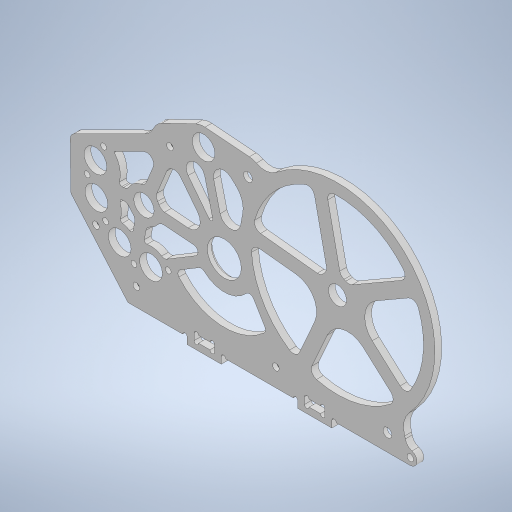
# Autodesk Inventor part: 右フレーム
Saved by Autodesk Inventor 2023 (Build 270158000, 158)
## iProperties
Created: 2022-06-19
Part Number: 右フレーム
Material: 一般
Document SubType Name: Modeling
Designer: muzho
Density: 1 g/cm^3
Appearance: 既定
Author: muzho
Autodesk Inventor part; units mm, degrees
ref_plane "YZ Plane" through (0, 0, 0) normal (1, 0, 0) x (0, 1, 0)
ref_plane "XZ Plane" through (0, 0, 0) normal (0, 1, 0) x (-1, 0, 0)
ref_plane "XY Plane" through (0, 0, 0) normal (0, 0, 1) x (1, 0, 0)
sketch "スケッチ1" plane through (0, 0, 0) normal (0, 0, 1) x (1, 0, 0)
  circle A0 centre (-51.0684, 48.1873) radius 1.3
  circle A1 centre (-58.3027, 33.9162) radius 1.3
  circle A2 centre (-50.1964, 20.1218) radius 1.3
  circle A3 centre (-37.7457, 10.0728) radius 1.3
  circle A4 centre (-22.565, 15.1272) radius 1.3
  circle A5 centre (-33.2954, 34.6933) radius 22.3153 construction
  circle A6 centre (2.1359, 32) radius 30.9835 construction
  circle A7 centre (52, 42.9528) radius 41.9528 construction
  circle A8 centre (2.1359, 32) radius 12.8528 construction
  circle A9 centre (-33.2954, 34.6933) radius 6.4335 construction
  circle A10 centre (-54.6856, 41.0518) radius 5.025
  circle A11 centre (-54.2496, 27.019) radius 5.025
  circle A12 centre (-43.9711, 15.0973) radius 5.025
  circle A13 centre (-30.1554, 12.6) radius 5.025
  circle A14 centre (-21.8214, 62.7533) radius 3
  circle A15 centre (-21.8214, 62.7533) radius 8
  line L0 (-21.8214, 62.7533) -> (-51.0684, 48.1873) construction
  line L1 (-33.3165, 55.1292) -> (-46.2281, 48.6988)
  arc A16 (-46.2281, 48.6988) -> (-46.7797, 47.8761) centre (-45.7823, 47.8037) ccw
  arc A17 (-52.9854, 52.0364) -> (-52.4722, 52.2518) centre (-51.0684, 48.1873) ccw construction
  arc A18 (-45.8061, 47.5867) -> (-65.5671, 39.279) centre (-54.6856, 41.0518) ccw construction
  line L2 (-65.7532, 43.7746) -> (-65.4452, 23.4769)
  arc A19 (-63.3575, 39.1831) -> (-63.6558, 28.9529) centre (-58.3027, 33.9162) ccw construction
  arc A20 (-45.2817, 33.4322) -> (-57.345, 16.4375) centre (-54.2496, 27.019) ccw construction
  arc A21 (-54.981, 15.674) -> (-41.5533, 4.3407) centre (-43.9711, 15.0973) ccw construction
  arc A22 (-65.4452, 23.4769) -> (-65.2027, 22.8391) centre (-64.4453, 23.4921) ccw
  line L3 (-65.2027, 22.8391) -> (-40.6377, -5.653)
  arc A23 (-40.6377, -5.653) -> (-39.8804, -6) centre (-39.8804, -5) ccw
  line L4 (-39.8804, -6) -> (84.0728, -6)
  line L5 (-6.7219, 36.0268) -> (-6.7219, -6.1434) construction
  line L6 (-37.0636, -3) -> (111.1776, -3) construction
  circle A24 centre (-10.2219, -3) radius 1
  circle A25 centre (-10.2219, -6) radius 1
  circle A26 centre (-15.2219, -6) radius 1
  line L7 (-11.2219, -3) -> (-11.2219, -6)
  circle A27 centre (-3.2219, -3) radius 1
  line L8 (-2.2219, -3) -> (-2.2219, -6)
  circle A28 centre (-3.2219, -6) radius 1
  circle A29 centre (1.7781, -6) radius 1
  line L9 (-9.2219, -3) -> (-4.2219, -3)
  line L10 (-14.2219, -6) -> (-14.2219, -9)
  line L11 (-14.2219, -9) -> (-7.7219, -9)
  line L12 (0.7781, -9) -> (-7.7219, -9)
  line L13 (0.7781, -6) -> (0.7781, -9)
  circle A30 centre (-33.2954, 34.6933) radius 4.5
  circle A31 centre (-33.2954, 34.6933) radius 7.5
  line L14 (-54.6856, 41.0518) -> (-54.2496, 27.019) construction
  line L15 (-54.4676, 34.0354) -> (-33.2954, 34.6933) construction
  arc A32 (-46.934, 49.3692) -> (-46.3247, 48.2383) centre (-44.0496, 50.1938) ccw
  arc A33 (-44.0483, 38.1537) -> (-46.3247, 48.2383) centre (-54.6856, 41.0518) ccw
  line L16 (-43.0524, 36.8913) -> (-42.313, 36.9143)
  line L17 (-42.8971, 31.8937) -> (-42.1577, 31.9167)
  arc A34 (-44.0483, 38.1537) -> (-43.0524, 36.8913) centre (-43.0835, 37.8908) ccw
  arc A35 (-42.8971, 31.8937) -> (-43.8127, 30.5719) centre (-42.8661, 30.8942) ccw
  arc A36 (-43.5733, 24.2678) -> (-43.8127, 30.5719) centre (-54.2496, 27.019) ccw
  arc A37 (-43.5733, 24.2678) -> (-42.7563, 23.0298) centre (-42.605, 24.0183) ccw
  arc A38 (-39.5768, 21.8123) -> (-42.7563, 23.0298) centre (-43.9711, 15.0973) ccw
  arc A39 (-42.313, 36.9143) -> (-39.8031, 38.4215) centre (-42.4062, 39.9128) ccw
  arc A40 (-39.5591, 30.5682) -> (-42.1577, 31.9167) centre (-42.0645, 28.9181) ccw
  arc A41 (-39.5768, 21.8123) -> (-38.0451, 22.4712) centre (-39.0292, 22.649) ccw
  line L18 (-38.0451, 22.4712) -> (-37.3465, 26.3363)
  line L19 (-43.9711, 15.0973) -> (-30.1554, 12.6) construction
  line L20 (-37.0632, 13.8486) -> (-33.2954, 34.6933) construction
  line L21 (-32.4262, 25.4469) -> (-33.1249, 21.5818)
  arc A42 (-33.1249, 21.5818) -> (-31.9208, 20.4284) centre (-32.1408, 21.4039) ccw
  arc A43 (-25.4967, 19.1343) -> (-31.9208, 20.4284) centre (-30.1554, 12.6) ccw
  arc A44 (-37.3465, 26.3363) -> (-38.2977, 29.1052) centre (-40.2986, 26.8699) ccw
  arc A45 (-30.5659, 27.7076) -> (-32.4262, 25.4469) centre (-29.4741, 24.9133) ccw
  arc A46 (-32.898, 62.0405) -> (-29.1429, 65.9774) centre (-36.4645, 69.2016) ccw
  line L22 (-21.8214, 62.7533) -> (-33.2954, 34.6933) construction
  line L23 (-29.2023, 51.3083) -> (-32.2241, 43.9183)
  line L24 (-23.2257, 52.7137) -> (-27.5961, 42.0259)
  arc A47 (-34.5136, 42.0937) -> (-32.2241, 43.9183) centre (-35.0009, 45.0538) ccw
  arc A48 (-27.5961, 42.0259) -> (-27.241, 39.1198) centre (-24.8193, 40.8904) ccw
  arc A49 (-29.2023, 51.3083) -> (-33.3165, 55.1292) centre (-31.9791, 52.4438) ccw
  circle A50 centre (2.1359, 32) radius 7.5
  circle A51 centre (2.1359, 32) radius 8.5
  arc A52 (-25.4967, 19.1343) -> (-23.3056, 19.0484) centre (-24.3356, 20.7628) ccw
  line L25 (-23.3056, 19.0484) -> (-10.3971, 26.8036)
  line L26 (-30.1554, 12.6) -> (2.1359, 32) construction
  arc A53 (-26.6272, 38.1263) -> (-24.1874, 36.5081) centre (-23.96, 39.4995) ccw
  arc A54 (-24.5663, 31.5225) -> (-27.2228, 30.2917) centre (-24.7937, 28.5311) ccw
  line L27 (-24.1874, 36.5081) -> (-13.7997, 35.7185)
  line L28 (-24.5663, 31.5225) -> (-11.2755, 30.5122)
  line L29 (-33.2954, 34.6933) -> (2.1359, 32) construction
  arc A55 (-10.3971, 26.8036) -> (-11.2755, 30.5122) centre (-11.4271, 28.518) ccw
  circle A56 centre (-54.6856, 41.0518) radius 14 construction
  line L30 (42, 44.1233) -> (42, -23.5713) construction
  circle A57 centre (38.5, -3) radius 1
  circle A58 centre (38.5, -6) radius 1
  circle A59 centre (33.5, -6) radius 1
  line L31 (37.5, -3) -> (37.5, -6)
  line L32 (34.5, -6) -> (34.5, -9)
  line L33 (34.5, -9) -> (42, -9)
  circle A60 centre (45.5, -3) radius 1
  line L34 (46.5, -3) -> (46.5, -6)
  circle A61 centre (45.5, -6) radius 1
  line L35 (49.5, -6) -> (49.5, -9)
  line L36 (49.5, -9) -> (42, -9)
  circle A62 centre (50.5, -6) radius 1
  line L37 (39.5, -3) -> (44.5, -3)
  circle A63 centre (52, 42.9528) radius 4.025
  circle A64 centre (52, 42.9528) radius 8.025
  arc A65 (83.7206, 13.9916) -> (24.9838, 76.3454) centre (52, 42.9528) ccw
  line L38 (52, 42.9528) -> (49.2725, 42.9528) construction
  arc A66 (55.6469, 50.1013) -> (58.5102, 50.1755) centre (57.0102, 52.7736) ccw
  line L39 (58.5102, 50.1755) -> (80.3207, 62.7679)
  arc A67 (80.3207, 62.7679) -> (81.1227, 67.2896) centre (78.8207, 65.3659) ccw
  arc A68 (61.5102, 44.9794) -> (60.0142, 42.5368) centre (63.0102, 42.3813) ccw
  arc A69 (87.6377, 56.0054) -> (83.3207, 57.5717) centre (84.8207, 54.9736) ccw
  line L40 (61.5102, 44.9794) -> (83.3207, 57.5717)
  line L41 (52, 42.9528) -> (85.5729, 62.3361) construction
  line L42 (52, 42.9528) -> (90.7666, 42.9528) construction
  line L43 (47.1425, 51.3763) -> (41.9063, 76.0106)
  arc A70 (46.3283, 48.6302) -> (47.1425, 51.3763) centre (44.2081, 50.7526) ccw
  arc A71 (41.9063, 76.0106) -> (37.8537, 78.1706) centre (38.9719, 75.3868) ccw
  arc A72 (50.5989, 80.8797) -> (47.7752, 77.258) centre (50.7097, 77.8818) ccw
  line L44 (53.0114, 52.6238) -> (47.7752, 77.258)
  arc A73 (53.0114, 52.6238) -> (54.8721, 50.4462) centre (55.9458, 53.2475) ccw
  line L45 (42.4877, 40.936) -> (17.4411, 43.5686)
  arc A74 (44.8478, 39.3131) -> (42.4877, 40.936) centre (42.1741, 37.9525) ccw
  arc A75 (17.4411, 43.5686) -> (14.1344, 40.3818) centre (17.1275, 40.585) ccw
  arc A76 (15.4964, 53.3403) -> (18.0683, 49.5357) centre (18.3818, 52.5193) ccw
  line L46 (43.1149, 46.9032) -> (18.0683, 49.5357)
  arc A77 (43.1149, 46.9032) -> (45.7609, 48) centre (43.4285, 49.8867) ccw
  line L47 (50.9786, 33.2829) -> (40.7351, 10.2756)
  arc A78 (53.2514, 35.026) -> (50.9786, 33.2829) centre (53.7192, 32.0627) ccw
  arc A79 (40.7351, 10.2756) -> (42.7441, 6.146) centre (43.4757, 9.0554) ccw
  arc A80 (30.8406, 11.4457) -> (35.2538, 12.716) centre (32.5132, 13.9362) ccw
  line L48 (45.4973, 35.7233) -> (35.2538, 12.716)
  arc A81 (45.4973, 35.7233) -> (45.2719, 38.5787) centre (42.7567, 36.9435) ccw
  line L49 (60.881, 38.9932) -> (79.5968, 22.1414)
  arc A82 (59.9256, 41.6934) -> (60.881, 38.9932) centre (62.8884, 41.2226) ccw
  arc A83 (79.5968, 22.1414) -> (84.1451, 22.776) centre (81.6042, 24.3708) ccw
  arc A84 (75.4264, 13.0928) -> (75.582, 17.6825) centre (73.5746, 15.4531) ccw
  line L50 (56.8662, 34.5343) -> (75.582, 17.6825)
  arc A85 (56.8662, 34.5343) -> (54.0809, 35.2023) centre (54.8588, 32.3049) ccw
  circle A86 centre (52, 42.9528) radius 37.9528
  circle A87 centre (-36.6731, 2) radius 1.5
  circle A88 centre (-36.6731, 2) radius 3
  line L51 (-39.8804, -5) -> (-36.6731, 2) construction
  circle A89 centre (24.8719, 2) radius 1.5
  circle A90 centre (24.8719, 2) radius 3
  line L52 (24.8719, 10.9511) -> (24.8719, -6.9511) construction
  circle A91 centre (84.0728, -3) radius 1.5
  circle A92 centre (84.0728, -3) radius 3
  circle A93 centre (-7, 69.8979) radius 5.025
  circle A94 centre (-7, 69.8979) radius 8
  line L53 (-10.4739, 77.1043) -> (-25.2953, 69.9597)
  arc A95 (-10.262, 60.4449) -> (-3.6097, 60.4901) centre (-7, 69.8979) ccw construction
  line L54 (-6.4881, 59.2404) -> (-2.9595, 44.6027)
  line L55 (-7, 69.8979) -> (2.1359, 32) construction
  line L56 (-2.5409, 59.9345) -> (0.2846, 48.214)
  arc A96 (-17.1837, 53.5456) -> (-23.2257, 52.7137) centre (-19.9638, 51.3798) ccw
  line L57 (-21.8214, 62.7533) -> (2.1359, 32) construction
  line L58 (-17.1837, 53.5456) -> (-9.516, 43.7028)
  arc A97 (-13.7997, 35.7185) -> (-9.516, 43.7028) centre (-13.4242, 40.6583) ccw
  line L59 (-13.8028, 55.7144) -> (-4.5495, 43.8363)
  arc A98 (-4.5495, 43.8363) -> (-2.9595, 44.6027) centre (-3.8372, 44.3911) ccw
  arc A99 (0.2846, 48.214) -> (9.4313, 48.6842) centre (4.8139, 49.3059) ccw
  arc A100 (10.184, 52.7694) -> (9.4313, 48.6842) centre (52, 42.9528) ccw
  arc A101 (-6.6918, 22.6584) -> (11.7715, 23.4941) centre (2.1359, 32) ccw
  arc A102 (-6.6918, 22.6584) -> (-9.0955, 22.9192) centre (-8.0655, 21.2048) ccw
  line L60 (-9.0955, 22.9192) -> (-17.3907, 17.9356)
  arc A103 (-17.3907, 17.9356) -> (-17.8823, 14.9232) centre (-16.3608, 16.2212) ccw
  arc A104 (-20.5941, 11.3055) -> (-18.526, 16.6024) centre (-22.565, 15.1272) ccw construction
  arc A105 (-17.8823, 14.9232) -> (19.613, 12.3302) centre (2.1359, 32) ccw
  arc A106 (14.9853, 23.2005) -> (11.7715, 23.4941) centre (13.2709, 22.1705) ccw
  line L61 (14.9853, 23.2005) -> (19.9989, 14.8552)
  arc A107 (19.613, 12.3302) -> (19.9989, 14.8552) centre (18.2846, 13.8252) ccw
  arc A108 (10.184, 52.7694) -> (7.1716, 62.4577) centre (0.4487, 55.0548) ccw
  arc A109 (16.2511, 75.4723) -> (24.9838, 76.3454) centre (19.952, 82.5648) ccw
  line L62 (-6.3807, 77.8739) -> (13.1663, 76.3562)
  line L63 (5.0173, 64.4141) -> (7.1716, 62.4577)
  arc A110 (-6.4881, 59.2404) -> (-13.8028, 55.7144) centre (-10.5261, 58.267) ccw
  arc A111 (5.0173, 64.4141) -> (-2.5409, 59.9345) centre (1.9273, 61.0116) ccw
  circle A112 centre (12.5499, 68.38) radius 4
  circle A113 centre (12.5499, 68.38) radius 8
  circle A114 centre (74.0428, 1.5165) radius 2
  arc A115 (76.7818, -6) -> (71.3037, -6) centre (74.0428, 1.5165) ccw
  arc A116 (83.7206, 13.9916) -> (81.6262, 4.0643) centre (91.1055, 7.2491) ccw
  arc A117 (81.8996, 3.0231) -> (84.8251, -0.0958) centre (85.8281, 3.7764) ccw
  arc A118 (-64.0909, 46.5055) -> (-65.7532, 43.7746) centre (-62.7535, 43.8201) ccw
  line L64 (-64.0909, 46.5055) -> (-32.898, 62.0405)
  circle A119 centre (2.1359, 32) radius 11.5
  circle A120 centre (74.0428, 1.5165) radius 3
  circle A121 centre (74.0428, 1.5165) radius 4
  circle A122 centre (12.5499, 68.38) radius 2
  circle A123 centre (-21.8214, 62.7533) radius 1.5
  circle A124 centre (-54.4309, 16.4709) radius 1.5
  circle A125 centre (-54.4309, 16.4709) radius 3
  arc A126 (-58.2926, 17.5135) -> (-53.5618, 12.5665) centre (-54.4309, 16.4709) ccw construction
  line L65 (-54.2496, 27.019) -> (-43.9711, 15.0973)
  line L66 (-54.4309, 16.4709) -> (-49.1103, 21.0581)
  arc A127 (68.9958, 49.3012) -> (67.3045, 33.2095) centre (73.9958, 40.6409) ccw
  arc A128 (63.2897, 28.7506) -> (47.4629, 25.3865) centre (56.5984, 21.3192) ccw
  arc A129 (41.9816, 27.827) -> (33.8915, 41.8396) centre (32.8462, 31.8943) ccw
  point P0 (0, 0)
  point P1 (0, 0)
  point P2 (29.8767, 73.7907)
  point P3 (16.7177, 56.9376)
  point P4 (46.0783, 56.3832)
  point P5 (-16.2219, -6)
  point P6 (0.7781, -6)
  point P7 (2.7781, -6)
  point P8 (32.5, -6)
  point P9 (51.5, -6)
  point P10 (-43.2615, 31.8127)
  point P11 (-43.4211, 36.9495)
  point P12 (-46.5149, 48.4843)
  point P13 (0.7781, -6)
  point P14 (-4.2219, -6)
  point P15 (-9.2219, -6)
  point P16 (44.5, -6)
  point P17 (39.5, -6)
  point P18 (81.3373, -1.7682)
  point P19 (54.8721, 50.4462)
  point P20 (50.5989, 80.8797)
  point P21 (15.4964, 53.3403)
  point P22 (14.1344, 40.3818)
  point P23 (44.8478, 39.3131)
  point P24 (45.2719, 38.5787)
  point P25 (30.8406, 11.4457)
  point P26 (42.7441, 6.146)
  point P27 (53.2514, 35.026)
  point P28 (54.0809, 35.2023)
  point P29 (75.4264, 13.0928)
  point P30 (84.1451, 22.776)
  point P31 (59.9256, 41.6934)
  point P32 (64.0505, 41.6862)
  point P33 (54.5192, 31.1007)
  point P34 (41.5064, 36.8943)
  point P35 (45.7609, 48)
  point P36 (46.3283, 48.6302)
  dimension "d19" = 3
  dimension "d21" = 2
  dimension "d22" = 2
  dimension "d59" = 2
  dimension "d60" = 2
  dimension "d2" = 10.05
  dimension "d3" = 10.05
  dimension "d4" = 10.05
  dimension "d5" = 10.05
  dimension "d6" = 6
  dimension "d7" = 16
  dimension "d8" = 1
  dimension "d9" = 3
  dimension "d10" = 6
  dimension "d11" = 6
  dimension "d12" = 6
  dimension "d13" = 1
  dimension "d14" = 6
  dimension "d15" = 1
  dimension "d16" = 6
  dimension "d17" = 35.4313
  dimension "d18" = 8.8578
  dimension "d20" = 2
  dimension "d23" = 5
  dimension "d24" = 3.5
  dimension "d25" = 3
  dimension "d26" = 9
  dimension "d27" = 3
  dimension "d28" = 3
  dimension "d29" = 5
  dimension "d30" = 2.5
  dimension "d31" = 1
  dimension "d32" = 1
  dimension "d33" = 3
  dimension "d34" = 1
  dimension "d35" = 3
  dimension "d36" = 3
  dimension "d37" = 1
  dimension "d38" = 1
  dimension "d39" = 3
  dimension "d40" = 5
  dimension "d41" = 2.5
  dimension "d42" = 3
  dimension "d43" = 3
  dimension "d44" = 8
  dimension "d45" = 3
  dimension "d46" = 3
  dimension "d47" = 5
  dimension "d48" = 2.5
  dimension "d49" = 3
  dimension "d50" = 15
  dimension "d51" = 2
  dimension "d52" = 2
  dimension "d53" = 3
  dimension "d54" = 3
  dimension "d55" = 5
  dimension "d56" = 2.5
  dimension "d57" = 2
  dimension "d58" = 2
  dimension "d61" = 3.5
  dimension "d62" = 5
  dimension "d63" = 3
  dimension "d64" = 8.05
  dimension "d65" = 4
  dimension "d66" = 1
  dimension "d67" = 3
  dimension "d68" = 3
  dimension "d69" = 3
  dimension "d70" = 30
  constraints: 180 point on circle, 130 end point, 120 centre point, 93 tangent, 24 coincident, 18 parallel, 16 concentric, 14 symmetric about line, 10 vertical, 4 horizontal, 4 midpoint, 4 point on line, 3 perpendicular, 2 equal radius, 2 vertical alignment, 1 equal length, 199 other
  measures "d2" diameter of A10
  measures "d3" diameter of A11
  measures "d4" diameter of A12
  measures "d5" diameter of A13
  measures "d6" diameter of A14
  measures "d7" diameter of A15
  measures "d8" radius of A16
  measures "d9" radial gap between concentric circles of A0 A17
  measures "d10" radial gap between concentric circles of A10 A18
  measures "d11" radial gap between concentric circles of A1 A19
  measures "d12" radial gap between concentric circles of A20 A11
  measures "d13" radius of A22
  measures "d14" radial gap between concentric circles of A21 A12
  measures "d15" radius of A23
  measures "d17" horizontal distance of point (2.136, 32) A5.centre
  measures "d18" distance from line of point (2.136, 32) L5
  measures "d20" diameter of A24
  measures "d23" distance of point (-10.222, -6) point (-15.222, -6)
  measures "d24" distance from line of L5 A24.centre
  measures "d25" distance of L10.start L10.end
  measures "d26" diameter of A30
  measures "d28" radius of A32
  measures "d29" distance between parallel lines of L17 L16
  measures "d30" distance between parallel lines of L17 L15
  measures "d31" radius of A34
  measures "d32" radius of A35
  measures "d33" radial gap between concentric circles of A12 A38
  measures "d34" radius of A37
  measures "d35" radius of A39
  measures "d36" radius of A40
  measures "d37" radius of A41
  measures "d38" radius of A42
  measures "d39" radial gap between concentric circles of A13 A43
  measures "d40" distance between parallel lines of L21 L18
  measures "d41" distance between parallel lines of L20 L21
  measures "d42" radius of A45
  measures "d43" radius of A44
  measures "d44" radius of A46
  measures "d45" radius of A47
  measures "d46" radius of A48
  measures "d47" distance between parallel lines of L24 L23
  measures "d48" distance between parallel lines of L24 L22
  measures "d49" radius of A49
  measures "d50" diameter of A50
  measures "d51" radius of A52
  measures "d52" distance between parallel lines of L26 L25
  measures "d53" radius of A53
  measures "d54" radius of A54
  measures "d55" distance between parallel lines of L28 L27
  measures "d56" distance between parallel lines of L28 L29
  measures "d57" radius of A55
  measures "d58" diameter of A57
  measures "d61" distance from line of L30 A57.centre
  measures "d62" distance of point (38.5, -6) point (33.5, -6)
  measures "d63" distance of L32.start L32.end
  measures "d64" diameter of A63
  measures "d65" radial gap between concentric circles of A63 A64
  measures "d67" radius of A66
  measures "d68" radius of A67
  measures "d69" radius of A68
  measures "d70" angle of L42 L41
extrude "押し出し1" add sketch "スケッチ1" against normal blind 3 contours A15 | A15 L53 A94 A110 | A110 L59 A98 L54 A94 A111 L56 A99 A100 A108 A113 A109 A65 A116 A115 L4 A62 L34 A60 L37 A57 L31 A59 A29 L8 A27 L9 A24 L7 A26 A23 L3 A22 L2 A118 L64 A46 A15 | A94 | L62 A113 L63 A111 A94 | A113 | A31 | A115 L4 | A117 A92 A115 | A92 | A92 L4 A115 | L4 A25 A28 L13 L12 L11 L10 | L35 L36 L33 L32 L4 A58 A61 | A64 | A64 A66 L39 A67 A86 A69 L40 A68 | A68 L40 A127 L49 A82 A64 | A64 A70 L43 A71 A86 A72 L44 A73 | A82 L49 A83 A86 A84 L50 A85 A64 | A85 L50 A128 L47 A78 A64 | A64 A74 L45 A75 A86 A76 L46 A77 | A78 L47 A79 A86 A80 L48 A81 A64 | A64 A81 L48 A129 L45 A74 | A119
extrude "押し出し2" add sketch "スケッチ1" against normal blind 1.8 contours A14 | A51 | A88 | A90 | A112 | A120 | A121 | A125
fillet "フィレット1" radius 1 1 edges at (70.0428, 1.5165, -1.8)
sketch "スケッチ2" plane through (0, 0, -3) normal (0, 0, -1) x (-1, 0, 0)
  arc A0 (-50.5989, 80.8797) -> (-81.1227, 67.2896) centre (-52, 42.9528) ccw projected
  arc A1 (-47.7752, 77.258) -> (-50.5989, 80.8797) centre (-50.7097, 77.8818) ccw projected
  line L0 (-47.7752, 77.258) -> (-53.0114, 52.6238) projected
  arc A2 (-54.8721, 50.4462) -> (-53.0114, 52.6238) centre (-55.9458, 53.2475) ccw projected
  arc A3 (-54.8721, 50.4462) -> (-55.6469, 50.1013) centre (-52, 42.9528) ccw projected
  arc A4 (-58.5102, 50.1755) -> (-55.6469, 50.1013) centre (-57.0102, 52.7736) ccw projected
  line L1 (-58.5102, 50.1755) -> (-80.3207, 62.7679) projected
  arc A5 (-81.1227, 67.2896) -> (-80.3207, 62.7679) centre (-78.8207, 65.3659) ccw projected
  circle A6 centre (-52, 42.9528) radius 4.025 projected
  circle A7 centre (-2.1359, 32) radius 8.5 projected
  arc A8 (2.5409, 59.9345) -> (-5.0173, 64.4141) centre (-1.9273, 61.0116) ccw projected
  line L2 (2.5409, 59.9345) -> (-0.2846, 48.214) projected
  arc A9 (-9.4313, 48.6842) -> (-0.2846, 48.214) centre (-4.8139, 49.3059) ccw projected
  arc A10 (-9.4313, 48.6842) -> (-10.184, 52.7694) centre (-52, 42.9528) ccw projected
  arc A11 (-7.1716, 62.4577) -> (-10.184, 52.7694) centre (-0.4487, 55.0548) ccw projected
  line L3 (-7.1716, 62.4577) -> (-5.0173, 64.4141) projected
  circle A12 centre (58.3027, 33.9162) radius 1.3 projected
  circle A13 centre (50.1964, 20.1218) radius 1.3 projected
  circle A14 centre (22.565, 15.1272) radius 1.3 projected
  circle A15 centre (54.6856, 41.0518) radius 5.025 projected
  circle A16 centre (30.1554, 12.6) radius 5.025 projected
  arc A17 (9.0955, 22.9192) -> (6.6918, 22.6584) centre (8.0655, 21.2048) ccw projected
  line L4 (9.0955, 22.9192) -> (17.3907, 17.9356) projected
  arc A18 (17.8823, 14.9232) -> (17.3907, 17.9356) centre (16.3608, 16.2212) ccw projected
  arc A19 (-19.613, 12.3302) -> (17.8823, 14.9232) centre (-2.1359, 32) ccw projected
  arc A20 (-19.9989, 14.8552) -> (-19.613, 12.3302) centre (-18.2846, 13.8252) ccw projected
  line L5 (-19.9989, 14.8552) -> (-14.9853, 23.2005) projected
  arc A21 (-11.7715, 23.4941) -> (-14.9853, 23.2005) centre (-13.2709, 22.1705) ccw projected
  arc A22 (-11.7715, 23.4941) -> (6.6918, 22.6584) centre (-2.1359, 32) ccw projected
  circle A23 centre (-24.8719, 2) radius 3 projected
  circle A24 centre (36.6731, 2) radius 3 projected
  circle A25 centre (37.7457, 10.0728) radius 1.3 projected
  circle A26 centre (51.0684, 48.1873) radius 1.3 projected
  line L6 (11.2219, -3) -> (11.2219, -6) projected
  arc A27 (9.2219, -6) -> (11.2219, -6) centre (10.2219, -6) ccw projected
  line L7 (9.2219, -6) -> (4.2219, -6) projected
  arc A28 (2.2219, -6) -> (4.2219, -6) centre (3.2219, -6) ccw projected
  line L8 (2.2219, -6) -> (2.2219, -3) projected
  arc A29 (4.2219, -3) -> (2.2219, -3) centre (3.2219, -3) ccw projected
  line L9 (4.2219, -3) -> (9.2219, -3) projected
  arc A30 (11.2219, -3) -> (9.2219, -3) centre (10.2219, -3) ccw projected
  line L10 (-37.5, -3) -> (-37.5, -6) projected
  arc A31 (-39.5, -6) -> (-37.5, -6) centre (-38.5, -6) ccw projected
  line L11 (-39.5, -6) -> (-44.5, -6) projected
  arc A32 (-46.5, -6) -> (-44.5, -6) centre (-45.5, -6) ccw projected
  line L12 (-46.5, -6) -> (-46.5, -3) projected
  arc A33 (-44.5, -3) -> (-46.5, -3) centre (-45.5, -3) ccw projected
  line L13 (-44.5, -3) -> (-39.5, -3) projected
  arc A34 (-37.5, -3) -> (-39.5, -3) centre (-38.5, -3) ccw projected
  circle A35 centre (33.2954, 34.6933) radius 4.5 projected
  circle A36 centre (21.8214, 62.7533) radius 3 projected
  circle A37 centre (-74.0428, 1.5165) radius 4 projected
  circle A38 centre (-12.5499, 68.38) radius 4 projected
  circle A39 centre (7, 69.8979) radius 5.025 projected
  arc A40 (27.241, 39.1198) -> (26.6272, 38.1263) centre (33.2954, 34.6933) ccw projected
  arc A41 (24.1874, 36.5081) -> (26.6272, 38.1263) centre (23.96, 39.4995) ccw projected
  line L14 (24.1874, 36.5081) -> (13.7997, 35.7185) projected
  arc A42 (9.516, 43.7028) -> (13.7997, 35.7185) centre (13.4242, 40.6583) ccw projected
  line L15 (9.516, 43.7028) -> (17.1837, 53.5456) projected
  arc A43 (23.2257, 52.7137) -> (17.1837, 53.5456) centre (19.9638, 51.3798) ccw projected
  line L16 (23.2257, 52.7137) -> (27.5961, 42.0259) projected
  arc A44 (27.241, 39.1198) -> (27.5961, 42.0259) centre (24.8193, 40.8904) ccw projected
  arc A45 (27.2228, 30.2917) -> (30.5659, 27.7076) centre (33.2954, 34.6933) ccw projected
  arc A46 (32.4262, 25.4469) -> (30.5659, 27.7076) centre (29.4741, 24.9133) ccw projected
  line L17 (32.4262, 25.4469) -> (33.1249, 21.5818) projected
  arc A47 (31.9208, 20.4284) -> (33.1249, 21.5818) centre (32.1408, 21.4039) ccw projected
  arc A48 (31.9208, 20.4284) -> (25.4967, 19.1343) centre (30.1554, 12.6) ccw projected
  arc A49 (23.3056, 19.0484) -> (25.4967, 19.1343) centre (24.3356, 20.7628) ccw projected
  line L18 (23.3056, 19.0484) -> (10.3971, 26.8036) projected
  arc A50 (11.2755, 30.5122) -> (10.3971, 26.8036) centre (11.4271, 28.518) ccw projected
  line L19 (11.2755, 30.5122) -> (24.5663, 31.5225) projected
  arc A51 (27.2228, 30.2917) -> (24.5663, 31.5225) centre (24.7937, 28.5311) ccw projected
  arc A52 (38.2977, 29.1052) -> (39.5591, 30.5682) centre (33.2954, 34.6933) ccw projected
  arc A53 (42.1577, 31.9167) -> (39.5591, 30.5682) centre (42.0645, 28.9181) ccw projected
  line L20 (42.1577, 31.9167) -> (42.8971, 31.8937) projected
  arc A54 (43.8127, 30.5719) -> (42.8971, 31.8937) centre (42.8661, 30.8942) ccw projected
  arc A55 (43.8127, 30.5719) -> (43.5733, 24.2678) centre (54.2496, 27.019) ccw projected
  arc A56 (42.7563, 23.0298) -> (43.5733, 24.2678) centre (42.605, 24.0183) ccw projected
  arc A57 (42.7563, 23.0298) -> (39.5768, 21.8123) centre (43.9711, 15.0973) ccw projected
  arc A58 (38.0451, 22.4712) -> (39.5768, 21.8123) centre (39.0292, 22.649) ccw projected
  line L21 (38.0451, 22.4712) -> (37.3465, 26.3363) projected
  arc A59 (38.2977, 29.1052) -> (37.3465, 26.3363) centre (40.2986, 26.8699) ccw projected
  arc A60 (39.8031, 38.4215) -> (42.313, 36.9143) centre (42.4062, 39.9128) ccw projected
  arc A61 (39.8031, 38.4215) -> (34.5136, 42.0937) centre (33.2954, 34.6933) ccw projected
  arc A62 (32.2241, 43.9183) -> (34.5136, 42.0937) centre (35.0009, 45.0538) ccw projected
  line L22 (32.2241, 43.9183) -> (29.2023, 51.3083) projected
  arc A63 (33.3165, 55.1292) -> (29.2023, 51.3083) centre (31.9791, 52.4438) ccw projected
  line L23 (33.3165, 55.1292) -> (46.2281, 48.6988) projected
  arc A64 (46.5149, 48.4843) -> (46.2281, 48.6988) centre (45.7823, 47.8037) ccw projected
  arc A65 (46.3247, 48.2383) -> (46.5149, 48.4843) centre (44.0496, 50.1938) ccw projected
  arc A66 (46.3247, 48.2383) -> (44.0483, 38.1537) centre (54.6856, 41.0518) ccw projected
  arc A67 (43.0524, 36.8913) -> (44.0483, 38.1537) centre (43.0835, 37.8908) ccw projected
  line L24 (43.0524, 36.8913) -> (42.313, 36.9143) projected
  circle A68 centre (43.9711, 15.0973) radius 5.025 projected
  circle A69 centre (54.2496, 27.019) radius 5.025 projected
  circle A70 centre (54.4309, 16.4709) radius 3 projected
  circle A71 centre (-84.0728, -3) radius 1.5 projected
  arc A72 (13.8028, 55.7144) -> (6.4881, 59.2404) centre (10.5261, 58.267) ccw projected
  line L25 (13.8028, 55.7144) -> (4.5495, 43.8363) projected
  arc A73 (2.9595, 44.6027) -> (4.5495, 43.8363) centre (3.8372, 44.3911) ccw projected
  line L26 (2.9595, 44.6027) -> (6.4881, 59.2404) projected
  arc A74 (29.1429, 65.9774) -> (32.898, 62.0405) centre (36.4645, 69.2016) ccw projected
  arc A75 (29.1429, 65.9774) -> (25.2953, 69.9597) centre (21.8214, 62.7533) ccw projected
  line L27 (25.2953, 69.9597) -> (10.4739, 77.1043) projected
  arc A76 (10.4739, 77.1043) -> (6.3807, 77.8739) centre (7, 69.8979) ccw projected
  line L28 (6.3807, 77.8739) -> (-13.1663, 76.3562) projected
  arc A77 (-13.1663, 76.3562) -> (-16.2511, 75.4723) centre (-12.5499, 68.38) ccw projected
  arc A78 (-24.9838, 76.3454) -> (-16.2511, 75.4723) centre (-19.952, 82.5648) ccw projected
  arc A79 (-24.9838, 76.3454) -> (-83.7206, 13.9916) centre (-52, 42.9528) ccw projected
  arc A80 (-81.6262, 4.0643) -> (-83.7206, 13.9916) centre (-91.1055, 7.2491) ccw projected
  arc A81 (-81.6262, 4.0643) -> (-81.8996, 3.0231) centre (-74.0428, 1.5165) ccw projected
  arc A82 (-84.8251, -0.0958) -> (-81.8996, 3.0231) centre (-85.8281, 3.7764) ccw projected
  arc A83 (-84.8251, -0.0958) -> (-84.0728, -6) centre (-84.0728, -3) ccw projected
  line L29 (-84.0728, -6) -> (-51.5, -6) projected
  arc A84 (-49.5, -6) -> (-51.5, -6) centre (-50.5, -6) ccw projected
  line L30 (-49.5, -6) -> (-49.5, -9) projected
  line L31 (-49.5, -9) -> (-34.5, -9) projected
  line L32 (-34.5, -9) -> (-34.5, -6) projected
  arc A85 (-32.5, -6) -> (-34.5, -6) centre (-33.5, -6) ccw projected
  line L33 (-32.5, -6) -> (-2.7781, -6) projected
  arc A86 (-0.7781, -6) -> (-2.7781, -6) centre (-1.7781, -6) ccw projected
  line L34 (-0.7781, -6) -> (-0.7781, -9) projected
  line L35 (-0.7781, -9) -> (14.2219, -9) projected
  line L36 (14.2219, -9) -> (14.2219, -6) projected
  arc A87 (16.2219, -6) -> (14.2219, -6) centre (15.2219, -6) ccw projected
  line L37 (16.2219, -6) -> (39.8804, -6) projected
  arc A88 (39.8804, -6) -> (40.6377, -5.653) centre (39.8804, -5) ccw projected
  line L38 (40.6377, -5.653) -> (65.2027, 22.8391) projected
  arc A89 (65.2027, 22.8391) -> (65.4452, 23.4769) centre (64.4453, 23.4921) ccw projected
  line L39 (65.4452, 23.4769) -> (65.7532, 43.7746) projected
  arc A90 (65.7532, 43.7746) -> (64.0909, 46.5055) centre (62.7535, 43.8201) ccw projected
  line L40 (64.0909, 46.5055) -> (32.898, 62.0405) projected
  arc A91 (-15.4964, 53.3403) -> (-37.8537, 78.1706) centre (-52, 42.9528) ccw projected
  arc A92 (-18.0683, 49.5357) -> (-15.4964, 53.3403) centre (-18.3818, 52.5193) ccw projected
  line L41 (-18.0683, 49.5357) -> (-43.1149, 46.9032) projected
  arc A93 (-45.7609, 48) -> (-43.1149, 46.9032) centre (-43.4285, 49.8867) ccw projected
  arc A94 (-45.7609, 48) -> (-46.3283, 48.6302) centre (-52, 42.9528) ccw projected
  arc A95 (-47.1425, 51.3763) -> (-46.3283, 48.6302) centre (-44.2081, 50.7526) ccw projected
  line L42 (-47.1425, 51.3763) -> (-41.9063, 76.0106) projected
  arc A96 (-37.8537, 78.1706) -> (-41.9063, 76.0106) centre (-38.9719, 75.3868) ccw projected
  arc A97 (-30.8406, 11.4457) -> (-14.1344, 40.3818) centre (-52, 42.9528) ccw projected
  arc A98 (-35.2538, 12.716) -> (-30.8406, 11.4457) centre (-32.5132, 13.9362) ccw projected
  line L43 (-35.2538, 12.716) -> (-41.9816, 27.827) projected
  arc A99 (-33.8915, 41.8396) -> (-41.9816, 27.827) centre (-32.8462, 31.8943) ccw projected
  line L44 (-33.8915, 41.8396) -> (-17.4411, 43.5686) projected
  arc A100 (-14.1344, 40.3818) -> (-17.4411, 43.5686) centre (-17.1275, 40.585) ccw projected
  arc A101 (-75.4264, 13.0928) -> (-42.7441, 6.146) centre (-52, 42.9528) ccw projected
  arc A102 (-75.582, 17.6825) -> (-75.4264, 13.0928) centre (-73.5746, 15.4531) ccw projected
  line L45 (-75.582, 17.6825) -> (-63.2897, 28.7506) projected
  arc A103 (-47.4629, 25.3865) -> (-63.2897, 28.7506) centre (-56.5984, 21.3192) ccw projected
  line L46 (-47.4629, 25.3865) -> (-40.7351, 10.2756) projected
  arc A104 (-42.7441, 6.146) -> (-40.7351, 10.2756) centre (-43.4757, 9.0554) ccw projected
  arc A105 (-84.1451, 22.776) -> (-79.5968, 22.1414) centre (-81.6042, 24.3708) ccw projected
  arc A106 (-87.6377, 56.0054) -> (-84.1451, 22.776) centre (-52, 42.9528) ccw projected
  arc A107 (-83.3207, 57.5717) -> (-87.6377, 56.0054) centre (-84.8207, 54.9736) ccw projected
  line L47 (-83.3207, 57.5717) -> (-68.9958, 49.3012) projected
  arc A108 (-67.3045, 33.2095) -> (-68.9958, 49.3012) centre (-73.9958, 40.6409) ccw projected
  line L48 (-67.3045, 33.2095) -> (-79.5968, 22.1414) projected
  point P0 (0, 0)
equation "\"d18\" = 0.25 * d17"
equation "\"d30\" = 0.5 * d29"
equation "\"d41\" = 0.5 * d40"
equation "\"d48\" = 0.5 * d47"
equation "\"d56\" = 0.5 * d55"
